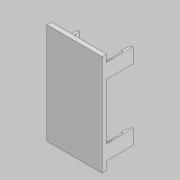
# Autodesk Inventor part: cover
Saved by Autodesk Inventor 2021.4 (Build 254397000, 397)
## iProperties
Created: 2022-11-07
Part Number: cover
Material: Generisch
Document SubType Name: Modeling
Designer: Tilman Preuschoff
Density: 1 g/cm^3
Appearance: Vorgabe
Author: Tilman Preuschoff
Autodesk Inventor part; units mm, degrees
ref_plane "YZ Plane" through (0, 0, 0) normal (1, 0, 0) x (0, 1, 0)
ref_plane "XZ Plane" through (0, 0, 0) normal (0, 1, 0) x (-1, 0, 0)
ref_plane "XY Plane" through (0, 0, 0) normal (0, 0, 1) x (1, 0, 0)
sketch "Skizze1" plane through (0, 0, 0) normal (0, 0, 1) x (1, 0, 0)
  line L0 (-12.5, 22.5) -> (12.5, 22.5)
  line L1 (12.5, 22.5) -> (12.5, -22.5)
  line L2 (12.5, -22.5) -> (-12.5, -22.5)
  line L3 (-12.5, -22.5) -> (-12.5, 22.5)
  line L4 (-12.5, 22.5) -> (12.5, -22.5) construction
  line L5 (12.5, 22.5) -> (-12.5, -22.5) construction
  point P0 (0, 0)
  dimension "d0" = 25
  dimension "d1" = 45
  constraints: 12 end point, 2 midpoint, 2 parallel, 1 horizontal, 1 perpendicular
  measures "d0" distance between parallel lines of L1 L3
  measures "d1" distance between parallel lines of L2 L0
extrude "Extrusion1" add sketch "Skizze1" along normal blind 2
sketch "Skizze3" plane through (0, 0, 0) normal (0, 0, -1) x (-1, 0, 0)
  line L0 (-12.5, -22.5) -> (-12.5, 22.5) projected
  line L1 (-12.5, -12.65) -> (-11.9, -12.65)
  line L2 (-11.9, -12.65) -> (-11.9, -19.35)
  line L3 (-11.9, -19.35) -> (-12.5, -19.35)
  line L4 (-12.5, -19.35) -> (-12.5, -12.65)
  line L5 (-12.5, 19.35) -> (-11.9, 19.35)
  line L6 (-11.9, 19.35) -> (-11.9, 12.65)
  line L7 (-11.9, 12.65) -> (-12.5, 12.65)
  line L8 (-12.5, 12.65) -> (-12.5, 19.35)
  line L9 (12.5, 22.5) -> (12.5, -22.5) projected
  line L10 (12.5, 13.35) -> (11.9, 13.35)
  line L11 (11.9, 13.35) -> (11.9, 6.65)
  line L12 (11.9, 6.65) -> (12.5, 6.65)
  line L13 (12.5, 6.65) -> (12.5, 13.35)
  line L14 (12.5, -12.65) -> (11.9, -12.65)
  line L15 (11.9, -12.65) -> (11.9, -19.35)
  line L16 (11.9, -19.35) -> (12.5, -19.35)
  line L17 (12.5, -19.35) -> (12.5, -12.65)
  line L18 (12.5, -22.5) -> (-12.5, -22.5) projected
  line L19 (-12.5, 22.5) -> (12.5, 22.5) projected
  point P0 (0, 0)
  dimension "d16" = 6.7
  dimension "d17" = 0.6
  dimension "d18" = 0.6
  dimension "d19" = 3.15
  dimension "d20" = 0.6
  dimension "d21" = 0.6
  dimension "d22" = 6.7
  dimension "d23" = 3.15
  dimension "d24" = 9.15
  dimension "d25" = 6.7
  constraints: 32 end point, 8 parallel, 6 point on line, 4 horizontal, 4 perpendicular
  measures "d16" distance between parallel lines of L3 L1
  measures "d17" distance between parallel lines of L0 L2
  measures "d18" distance between parallel lines of L9 L15
  measures "d19" distance between parallel lines of L3 L18
  measures "d20" distance between parallel lines of L6 L0
  measures "d21" distance between parallel lines of L9 L11
  measures "d22" distance between parallel lines of L7 L5
  measures "d23" distance between parallel lines of L5 L19
  measures "d24" distance between parallel lines of L10 L19
  measures "d25" distance between parallel lines of L10 L12
extrude "Extrusion2" add sketch "Skizze3" along normal blind 8 contours L0 L1 L2 L3 | L16 L15 L14 L9 | L0 L5 L6 L7 | L12 L11 L10 L9
sketch "Skizze4" plane through (11.9, -19.35, 0) normal (0, -1, 0) x (1, 0, 0)
  line L0 (0.6, 0) -> (0.6, -8) projected
  line L1 (0.6, -8) -> (-0.55, -8)
  line L2 (-0.55, -8) -> (-0.55, -12)
  line L3 (-0.55, -12) -> (0.6, -12)
  line L4 (0.6, -12) -> (0.6, -8)
  line L5 (-24.4, 0) -> (-24.4, -8) projected
  line L6 (-24.4, -8) -> (-23.25, -8)
  line L7 (-23.25, -8) -> (-23.25, -12)
  line L8 (-23.25, -12) -> (-24.4, -12)
  line L9 (-24.4, -12) -> (-24.4, -8)
  line L10 (-0.55, -10) -> (0.025, -12)
  line L11 (-23.25, -10) -> (-23.825, -12)
  point P0 (-11.9, 0)
  dimension "d28" = 1.15
  dimension "d29" = 1.15
  dimension "d30" = 4
  dimension "d31" = 4
  constraints: 20 end point, 4 midpoint, 4 parallel, 2 horizontal, 2 perpendicular
  measures "d28" distance between parallel lines of L2 L4
  measures "d29" distance between parallel lines of L9 L7
  measures "d30" distance between parallel lines of L1 L3
  measures "d31" distance between parallel lines of L6 L8
extrude "Extrusion3" add sketch "Skizze4" against normal up to surface (6.7 mm away) contours L4 L3 L10 L2 L1 | L6 L7 L11 L8 L9
sketch "Skizze6" plane through (-12.5, 6.65, 0) normal (0, -1, 0) x (1, 0, 0)
  line L0 (0, -8) -> (1.15, -8)
  line L1 (1.15, -8) -> (1.15, -12)
  line L2 (1.15, -12) -> (0, -12)
  line L3 (0, -12) -> (0, -8)
  line L4 (1.15, -10) -> (0.575, -12)
  point P0 (12.5, 0)
  dimension "d36" = 1.15
  dimension "d37" = 4
  constraints: 10 end point, 2 midpoint, 2 parallel, 1 coincident, 1 horizontal, 1 perpendicular
  measures "d36" distance between parallel lines of L3 L1
  measures "d37" distance between parallel lines of L0 L2
extrude "Extrusion4" add sketch "Skizze6" against normal up to surface (6.7 mm away) contours L0 L1 L4 L2 L3
sketch "Skizze7" plane through (11.9, 12.65, 0) normal (0, -1, 0) x (1, 0, 0)
  line L0 (0.6, -8) -> (-0.55, -8)
  line L1 (-0.55, -8) -> (-0.55, -12)
  line L2 (-0.55, -12) -> (0.6, -12)
  line L3 (0.6, -12) -> (0.6, -8)
  line L4 (-0.55, -10) -> (0.025, -12)
  point P0 (-11.9, 0)
  dimension "d40" = 1.15
  dimension "d41" = 4
  constraints: 10 end point, 2 midpoint, 2 parallel, 1 coincident, 1 horizontal, 1 perpendicular
  measures "d40" distance between parallel lines of L1 L3
  measures "d41" distance between parallel lines of L0 L2
extrude "Extrusion5" add sketch "Skizze7" against normal up to surface (6.7 mm away) contours L3 L2 L4 L1 L0
sketch "Skizze8" plane through (-12.5, -22.5, 0) normal (0, -1, 0) x (1, 0, 0)
  line L0 (25, 0) -> (24.4, 0) projected
  line L1 (25, 2) -> (0, 2) projected
  line L2 (25, 0) -> (0, 0)
  line L3 (0, 0) -> (0, 2)
  line L4 (0, 2) -> (25, 2)
  line L5 (25, 2) -> (25, 0)
  point P0 (12.5, 0)
  constraints: 8 end point, 2 parallel, 1 horizontal, 1 perpendicular
extrude "Extrusion6" add sketch "Skizze8" along normal blind 0.7
